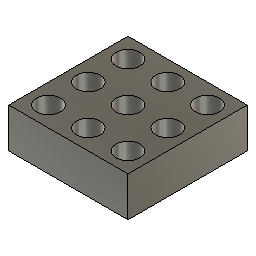
Nozzle Holder (Autodesk Fusion 360 design; units mm, degrees)
Autodesk Fusion 360 part; units mm, degrees
sketch "Sketch1" plane through (0, 0, 0) normal (0, 0, 1) x (1, 0, 0)
  circle A0 centre (0, 0) radius 3
  circle A1 centre (10, 0) radius 3
  circle A2 centre (20, 0) radius 3
  circle A3 centre (0, 10) radius 3
  circle A4 centre (20, 10) radius 3
  circle A5 centre (10, 10) radius 3
  circle A6 centre (0, 20) radius 3
  circle A7 centre (20, 20) radius 3
  circle A8 centre (10, 20) radius 3
  line L0 (25, 25) -> (-5, 25)
  line L1 (-5, 25) -> (-5, -5)
  line L2 (-5, -5) -> (25, -5)
  line L3 (25, -5) -> (25, 25)
  line L4 (25, 25) -> (-5, -5) construction
  line L5 (-5, 25) -> (25, -5) construction
  point P0 (10, 10)
  dimension "d1" = 6
  dimension "d4" = 20
  dimension "d5" = 0
  dimension "d8" = 0
  dimension "d9" = 20
  dimension "d10" = 30
  dimension "d11" = 30
  constraint coincident A0.centre origin
  constraint horizontal L0
  constraint perpendicular L0 L1
  constraint parallel L0 L2
  constraint parallel L1 L3
  constraint coincident L4 P0
  constraint coincident L5 P0
  constraint coincident P0 A5.centre
  measures "d1" diameter of A0
  measures "d10" distance of L1.end L2.end
  measures "d11" distance of L0.end L1.end
extrude "Extrude1" add sketch "Sketch1" along normal blind 10
